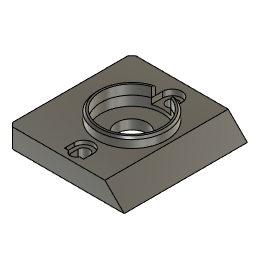
Z#bearing_holder (Autodesk Fusion 360 design; units mm, degrees)
Autodesk Fusion 360 part; units mm, degrees
sketch "Sketch1" plane through (0, 0, 0) normal (0, 0, 1) x (1, 0, 0)
  line L0 (0, 0) -> (30, 0)
  line L1 (30, 0) -> (30, 35)
  line L2 (30, 35) -> (0, 35)
  line L3 (0, 35) -> (0, 0)
  dimension "d1" = 30
  dimension "d2" = 35
  constraint horizontal L0
  constraint vertical L1
  constraint horizontal L2
  constraint vertical L3
  constraint coincident L0.start L3.end
  measures "d1" distance of L0.start L0.end
  measures "d2" distance of L0.start L2.end
extrude "Extrude1" add sketch "Sketch1" along normal blind 5 makes body 1
sketch "Sketch2" plane through (0, 0, 5) normal (0, 0, 1) x (-1, 0, 0)
  line L0 (0, -35) -> (0, 0)
  line L1 (0, 0) -> (-30, 0)
  line L2 (-30, 0) -> (-30, -35)
  line L3 (-30, -35) -> (0, -35)
  line L4 (-30, -17.5) -> (-15, -17.5)
  circle A0 centre (-15, -17.5) radius 4
  line L5 (-15, -13.5) -> (-15, -6.5)
  line L6 (-15, -21.5) -> (-15, -26.5)
  line L7 (-15, -26.5) -> (-15, -28)
  circle A1 centre (-15, -28) radius 1.5
  line L8 (-15, -6.5) -> (-15, -5)
  circle A2 centre (-15, -5) radius 1.5
  circle A3 centre (-15, -17.5) radius 8
  circle A4 centre (-15, -17.5) radius 9
  circle A5 centre (-15, -28) radius 2.5
  circle A6 centre (-15, -5) radius 2.5
  dimension "d5" = 8
  dimension "d6" = 7
  dimension "d7" = 5
  dimension "d8" = 1.5
  dimension "d9" = 3
  dimension "d10" = 1.5
  dimension "d11" = 16
  dimension "d12" = 18
  dimension "d13" = 5
  dimension "d14" = 5
  constraint midpoint L2 L4.start
  constraint perpendicular L2 L4
  constraint coincident L4.end A0.centre
  constraint coincident A0 L5.start
  constraint perpendicular L4 L5
  constraint coincident A0 L6.start
  constraint perpendicular L4 L6
  constraint vertical L7
  constraint coincident L7.end A1.centre
  constraint parallel L5 L8
  constraint coincident L8.end A2.centre
  constraint coincident L5.end A2
  constraint concentric A0 A3
  constraint concentric A0 A4
  constraint concentric A1 A5
  constraint concentric A2 A6
  measures "d5" diameter of A0
  measures "d6" distance of L5.start L5.end
  measures "d7" distance of L6.start L6.end
  measures "d8" distance of L6.end L7.end
  measures "d9" diameter of A1
  measures "d10" distance of L5.end L8.end
  measures "d11" diameter of A3
  measures "d12" diameter of A4
  measures "d13" diameter of A5
  measures "d14" diameter of A6
extrude "Extrude2" cut sketch "Sketch2" against normal blind 5 contours A1 | A2 bodies 1
extrude "Extrude3" cut sketch "Sketch2" against normal blind 3 contours A6 bodies 1
extrude "Extrude4" cut sketch "Sketch2" against normal blind 3 contours L6 A4 A5 | A4 A5 | L6 A4 A5 bodies 1
extrude "Extrude5" add sketch "Sketch2" along normal blind 2.5 separate body contours L4 L5 A3 A4 | L4 A3 A4 A5 | L5 A3 A4 A5 makes body 2
extrude "Extrude6" cut sketch "Sketch2" against normal blind 2.5 contours L4 A0 L5 A3 | L4 A0 L6 A3 | A0 | A0 L5 L6 A3 bodies 1
extrude "Extrude7" cut sketch "Sketch2" against normal blind 50 contours A0 bodies 1
extrude "Extrude8" cut 1 faces at (10, 0, 1.6667) along direction (0, 1, 0) blind 0.5 on bodies 1 bodies 1
extrude "Extrude9" cut 1 faces at (20, 35, 1.6667) along direction (0, -1, 0) blind 0.5 on bodies 1 bodies 1
chamfer "Chamfer1" distance 5 angle 45 1 edges at (30, 17.5, 5) on bodies 1
extrude "Extrude10" add 1 faces at (12.8482, 27.8013, 2) along direction (0, 0, 1) blind 1.5 on bodies 1 bodies 1
extrude "Extrude11" add 1 faces at (12.8482, 4.8013, 2) along direction (0, 0, 1) blind 1.5 on bodies 1 bodies 1
chamfer "Chamfer2" distance 1 angle 45 1 edges at (0, 34.5, 2.5) on bodies 1
chamfer "Chamfer3" distance 1 angle 45 1 edges at (0, 0.5, 2.5) on bodies 1
chamfer "Chamfer4" distance 0.5 angle 45 1 edges at (15, 8.5, 7.5) on bodies 2
sketch "Sketch3" plane through (0, 0, 5) normal (0, 0, 1) x (-1, 0, 0)
  circle A0 centre (-15, -28) radius 2.5
  circle A1 centre (-15, -17.5) radius 8
  circle A2 centre (-15, -5) radius 2.5
  line L0 (0, -1.5) -> (-1, -0.5)
  line L1 (-1, -0.5) -> (-25, -0.5)
  line L2 (-25, -0.5) -> (-25, -34.5)
  line L3 (-25, -34.5) -> (-1, -34.5)
  line L4 (-1, -34.5) -> (0, -33.5)
  line L5 (0, -33.5) -> (0, -1.5)
  line L6 (-15, -28) -> (-12.5, -28)
  line L7 (-12.5, -28) -> (-12.5, -25.0993)
  line L8 (-15, -28) -> (-17.5, -28)
  line L9 (-17.5, -28) -> (-17.5, -25)
  line L10 (-17.5, -25) -> (-12.5, -25.0993)
  constraint coincident A0.centre L6.start
  constraint coincident A0 L6.end
  constraint horizontal L6
  constraint coincident A1 L7.end
  constraint tangent A0 L7
  constraint coincident A0 L8.end
  constraint parallel L6 L8
  constraint tangent A0 L9
extrude "Extrude12" cut sketch "Sketch3" along normal blind 3.9 contours A0 A1 L9 | A0 A1 L7 bodies 2
extrude "Extrude13" cut sketch "Sketch3" against normal blind 1.5 contours A0 A1 L9 | A0 A1 L7 bodies 1
extrude "Extrude14" cut 1 faces at (18.667, 34.5, 1.6667) along direction (0, -1, 0) blind 2 on bodies 1 bodies 1
extrude "Extrude15" cut 1 faces at (1, 33.8333, 1.6667) along direction (-1, 0, 0) blind 7 on bodies 1 bodies 1
chamfer "Chamfer5" distance 1 angle 45 1 edges at (0, 32.5, 2.5) on bodies 1
sketch "Sketch4" plane through (0, 0, 5) normal (0, 0, 1) x (-1, 0, 0)
  line L0 (-17.5, -28) -> (-17.5, -25.0993)
  arc A0 (-12.5, -25.0993) -> (-17.5, -25.0993) centre (-15, -17.5) ccw
  line L1 (-12.5, -25.0993) -> (-12.5, -28)
  arc A1 (-17.5, -28) -> (-12.5, -28) centre (-15, -28) ccw
  circle A2 centre (-15, -5) radius 2.5
  line L2 (-1, -32.5) -> (0, -31.5)
  line L3 (0, -31.5) -> (0, -1.5)
  line L4 (0, -1.5) -> (-1, -0.5)
  line L5 (-1, -0.5) -> (-25, -0.5)
  line L6 (-25, -0.5) -> (-25, -32.5)
  line L7 (-25, -32.5) -> (-1, -32.5)
  line L8 (-12.5, -5) -> (-12.5, -3)
  arc A3 (-12.5, -3) -> (-17.5, -3) centre (-15, -3) ccw
  line L9 (-17.5, -3) -> (-17.5, -5)
  arc A4 (-17.5, -5) -> (-12.5, -5) centre (-15, -5) ccw
  line L10 (-15, -5) -> (-15, -3) construction
  constraint tangent L8 A3
  constraint tangent A3 L9
  constraint parallel L8 L9
  constraint tangent L9 A4
  constraint tangent L8 A4
  constraint vertical L10
  constraint coincident A2.centre A4.centre
extrude "Extrude16" cut sketch "Sketch4" against normal blind 2 contours A2 L8 A3 L9 bodies 1
extrude "Extrude17" add 1 faces at (15, 1.838, 3) along direction (0, 0, 1) blind 0.5 on bodies 1 bodies 1
sketch "Sketch5" plane through (0, 0, 3.5) normal (0, 0, 1) x (-1, 0, 0)
  circle A0 centre (-15, -5) radius 1.5
  arc A1 (-17.5, -5) -> (-12.5, -5) centre (-15, -5) ccw
  line L0 (-12.5, -5) -> (-12.5, -3)
  arc A2 (-12.5, -3) -> (-15, -0.5) centre (-15, -3) ccw
  arc A3 (-15, -0.5) -> (-17.5, -3) centre (-15, -3) ccw
  line L1 (-17.5, -3) -> (-17.5, -5)
  line L2 (-15, -0.5) -> (-15, -1.5)
  circle A4 centre (-15, -3) radius 1.5
  line L3 (-13.5, -3) -> (-13.5, -5.2)
  line L4 (-13.5, -5.2) -> (-16.4866, -5.2)
  line L5 (-16.4866, -2.8) -> (-16.4866, -5.2)
  constraint coincident A2.end A3.start
  constraint vertical L2
  constraint concentric A2 A4
  constraint coincident L2.end A4
  constraint coincident A4 L3.start
  constraint tangent A4 L3
  constraint vertical L3
  constraint coincident A0 L4.end
  constraint perpendicular L3 L4
  constraint coincident A4 L5.start
  constraint perpendicular L4 L5
extrude "Extrude18" cut sketch "Sketch5" against normal blind 5 contours A0 A4 L4 L5 | A0 A4 L3 | A0 A4 | A0 A4 L5 | A0 A4 L5 bodies 1
sketch "Sketch6" plane through (0, 0, 5) normal (0, 0, 1) x (-1, 0, 0)
  line L0 (-12.5, -3) -> (-12.5, -5)
  arc A0 (-17.5, -5) -> (-12.5, -5) centre (-15, -5) ccw
  line L1 (-17.5, -5) -> (-17.5, -3)
  arc A1 (-15, -0.5) -> (-17.5, -3) centre (-15, -3) ccw
  line L2 (-15, -0.5) -> (-25, -0.5)
  line L3 (-25, -0.5) -> (-25, -32.5)
  line L4 (-25, -32.5) -> (-1, -32.5)
  line L5 (-1, -32.5) -> (0, -31.5)
  line L6 (0, -31.5) -> (0, -1.5)
  line L7 (0, -1.5) -> (-1, -0.5)
  line L8 (-1, -0.5) -> (-15, -0.5)
  arc A2 (-12.5, -3) -> (-15, -0.5) centre (-15, -3) ccw
  line L9 (-17.5, -28) -> (-17.5, -25.0993)
  arc A3 (-12.5, -25.0993) -> (-17.5, -25.0993) centre (-15, -17.5) ccw
  line L10 (-12.5, -25.0993) -> (-12.5, -28)
  arc A4 (-17.5, -28) -> (-12.5, -28) centre (-15, -28) ccw
  line L11 (-11.4497, -0.5) -> (-19.5, -0.5)
  line L12 (-19.5, -0.5) -> (-19.5, -2.5)
  line L13 (-19.5, -2.5) -> (-11.4497, -2.5)
  line L14 (-11.4497, -2.5) -> (-11.4497, -0.5)
  constraint horizontal L11
  constraint vertical L12
  constraint horizontal L13
  constraint vertical L14
  constraint coincident L8 L11.start
extrude "Extrude19" add 1 faces at (16.8244, 3.5333, 3.5) along direction (0, 0, 1) blind 5.5 on bodies 1 bodies 1
extrude "Extrude20" cut 1 faces at (16.8244, 3.5333, 9) along direction (0, 0, -1) blind 4 on bodies 1 bodies 1
extrude "Extrude21" cut sketch "Sketch6" against normal blind 1 contours L0 A0 L1 A1 A2 L13 bodies 1
